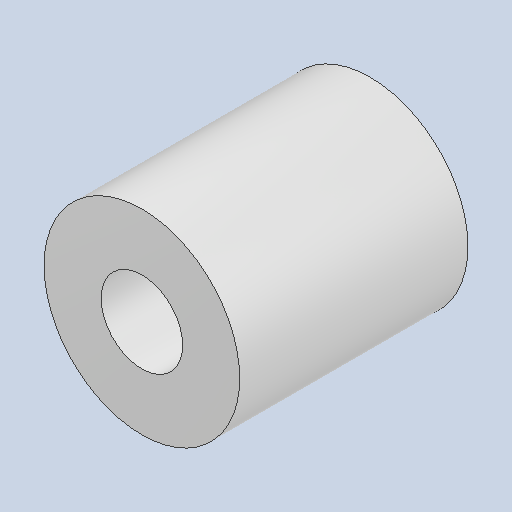
# Autodesk Inventor part: l40
Saved by Autodesk Inventor 2023 (Build 270158000, 158)
## iProperties
Created: 2022-01-09
Part Number: l40
Material: Aluminum 2014-T4
Document SubType Name: Modeling
Designer: acps
Density: 2.8 g/cm^3
Appearance: Satin
Author: acps
Autodesk Inventor part; units mm, degrees
ref_plane "YZ Plane" through (0, 0, 0) normal (1, 0, 0) x (0, 1, 0)
ref_plane "XZ Plane" through (0, 0, 0) normal (0, 1, 0) x (-1, 0, 0)
ref_plane "XY Plane" through (0, 0, 0) normal (0, 0, 1) x (1, 0, 0)
sketch "Sketch1" plane through (0, 0, 0) normal (0, 0, 1) x (1, 0, 0)
  circle A0 centre (0, 0) radius 1.25
  circle A1 centre (0, 0) radius 3
  dimension "d0" = 2.5
  dimension "d1" = 6
  constraints: 2 centre point, 2 coincident
  measures "d0" diameter of A0
  measures "d1" diameter of A1
extrude "Extrusion1" add sketch "Sketch1" against normal blind 7
body "Solid1"
